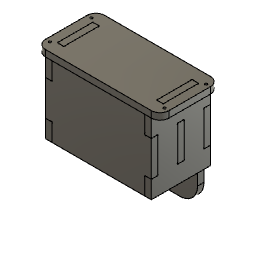
ArmorToolPocketHoleStation v2 (Autodesk Fusion 360 design; units mm, degrees)
Autodesk Fusion 360 part; units mm, degrees
sketch "Sketch1" plane through (0, 0, 0) normal (0, 1, 0) x (1, 0, 0)
  line L0 (0, 0) -> (266.7, 0)
  line L1 (266.7, 0) -> (266.7, -18.542)
  line L2 (266.7, -18.542) -> (0, -18.542)
  line L3 (0, -18.542) -> (0, 0)
  dimension "d1" = 266.7
  dimension "d2" = 18.542
  constraint horizontal L0
  constraint vertical L1
  constraint horizontal L2
  constraint vertical L3
  constraint coincident L0.start L3.end
  measures "d1" distance of L0.start L0.end
  measures "d2" distance of L0.start L2.end
extrude "Extrude1" add sketch "Sketch1" along normal blind 203.2 makes body 1 in component "Component"
sketch "Sketch2" plane through (0, 0, 18.542) normal (0, 0, 1) x (1, 0, 0)
  line L0 (0, 0) -> (266.7, 0)
  line L1 (266.7, 0) -> (266.7, 203.2)
  line L2 (266.7, 203.2) -> (0, 203.2)
  line L3 (0, 203.2) -> (0, 0)
  line L4 (0, 203.2) -> (0, 152.4) construction
  line L5 (266.7, 203.2) -> (266.7, 152.4) construction
  line L6 (0, 152.4) -> (-18.542, 152.4)
  line L7 (-18.542, 152.4) -> (-18.542, 50.8)
  line L8 (-18.542, 50.8) -> (0, 50.8)
  line L9 (0, 50.8) -> (0, 152.4)
  line L10 (266.7, 152.4) -> (285.242, 152.4)
  line L11 (285.242, 152.4) -> (285.242, 50.8)
  line L12 (285.242, 50.8) -> (266.7, 50.8)
  line L13 (266.7, 50.8) -> (266.7, 152.4)
  dimension "d5" = 50.8
  dimension "d7" = 50.8
  dimension "d8" = 18.542
  dimension "d9" = 101.6
  dimension "d10" = 18.542
  dimension "d11" = 101.6
  constraint coincident L2.end L3.start
  constraint perpendicular L2 L4
  constraint coincident L1.end L2.start
  constraint perpendicular L2 L5
  constraint horizontal L6
  constraint vertical L7
  constraint horizontal L8
  constraint vertical L9
  constraint horizontal L10
  constraint vertical L11
  constraint horizontal L12
  constraint vertical L13
  measures "d5" distance of L2.end L4.end
  measures "d7" distance of L1.end L5.end
  measures "d8" distance of L4.end L6.end
  measures "d9" distance of L4.end L8.end
  measures "d10" distance of L5.end L10.end
  measures "d11" distance of L5.end L12.end
extrude "Extrude2" add sketch "Sketch2" against normal up to surface (18.542 mm away) contours L3 L6 L7 L8 L9 | L1 L10 L11 L12 L13 bodies 1 in component "Component"
sketch "Sketch3" plane through (0, 0, 0) normal (-1, 0, 0) x (0, 0, 1)
  line L0 (0, 152.4) -> (18.542, 152.4)
  line L1 (18.542, 152.4) -> (18.542, 50.8)
  line L2 (18.542, 50.8) -> (0, 50.8)
  line L3 (0, 50.8) -> (0, 152.4)
  line L4 (94.234, 203.2) -> (94.234, 152.4)
  line L5 (94.234, 152.4) -> (75.692, 152.4)
  line L6 (75.692, 152.4) -> (75.692, 50.8)
  line L7 (75.692, 50.8) -> (94.234, 50.8)
  line L8 (94.234, 50.8) -> (94.234, 0)
  line L9 (94.234, 0) -> (-75.692, 0)
  line L10 (-75.692, 0) -> (-75.692, 50.8)
  line L11 (-75.692, 50.8) -> (-57.15, 50.8)
  line L12 (-57.15, 50.8) -> (-57.15, 152.4)
  line L13 (-57.15, 152.4) -> (-75.692, 152.4)
  line L14 (-75.692, 152.4) -> (-75.692, 203.2)
  line L15 (-75.692, 203.2) -> (94.234, 203.2)
  dimension "d15" = 50.8
  dimension "d16" = 18.542
  dimension "d17" = 101.6
  dimension "d18" = 18.542
  dimension "d19" = 169.926
  dimension "d20" = 18.542
  dimension "d21" = 101.6
  constraint coincident L0.end L1.start
  constraint perpendicular L0 L1
  constraint perpendicular L1 L2
  constraint coincident L0.start L3.end
  constraint perpendicular L0 L3
  constraint perpendicular L4 L5
  constraint perpendicular L5 L6
  constraint perpendicular L6 L7
  constraint perpendicular L7 L8
  constraint perpendicular L8 L9
  constraint perpendicular L9 L10
  constraint perpendicular L10 L11
  constraint perpendicular L9 L12
  constraint perpendicular L3 L13
  constraint perpendicular L13 L14
  measures "d15" distance of L4.start L4.end
  measures "d16" distance of L4.end L5.end
  measures "d17" distance of L5.end L6.end
  measures "d18" distance of L6.end L7.end
  measures "d19" distance of L8.end L9.end
  measures "d20" distance of L10.end L11.end
  measures "d21" distance of L11.end L12.end
extrude "Extrude1'" add sketch "Sketch3" along normal blind 18.542 separate body makes body 2 in component "Component'"
sketch "Sketch4" plane through (0, 0, -57.15) normal (0, 0, -1) x (-1, 0, 0)
  line L0 (0, 50.8) -> (18.542, 50.8)
  line L1 (18.542, 50.8) -> (18.542, 152.4)
  line L2 (18.542, 152.4) -> (0, 152.4)
  line L3 (0, 50.8) -> (0, -101.6)
  line L4 (0, -101.6) -> (-266.7, -101.6)
  line L5 (-266.7, -101.6) -> (-266.7, 50.8)
  line L6 (-266.7, 50.8) -> (-285.242, 50.8)
  line L7 (-285.242, 50.8) -> (-285.242, 152.4)
  line L8 (-285.242, 152.4) -> (-266.7, 152.4)
  line L9 (-266.7, 152.4) -> (-266.7, 203.2)
  line L10 (-266.7, 203.2) -> (0, 203.2)
  line L11 (0, 203.2) -> (0, 152.4)
  dimension "d24" = 152.4
  dimension "d25" = 266.7
  dimension "d26" = 18.542
  constraint coincident L0.start L3.start
  constraint perpendicular L0 L3
  constraint perpendicular L3 L4
  constraint perpendicular L4 L5
  constraint perpendicular L5 L6
  constraint perpendicular L6 L7
  constraint perpendicular L7 L8
  constraint perpendicular L8 L9
  constraint perpendicular L9 L10
  constraint coincident L2.end L11.end
  constraint perpendicular L2 L11
  measures "d24" distance of L0.start L3.end
  measures "d25" distance of L3.end L4.end
  measures "d26" distance of L5.end L6.end
extrude "Extrude1''" add sketch "Sketch4" along normal blind 18.542 separate body makes body 3 in component "Component''"
fillet "Fillet1" radius 50.8 2 edges at (266.7, -101.6, -66.421) (0, -101.6, -66.421) on bodies 3 in component "Component''"
sketch "Sketch5" plane through (-18.542, 0, 0) normal (-1, 0, 0) x (0, 0, 1)
  line L0 (18.542, 50.8) -> (0, 50.8)
  line L1 (0, 50.8) -> (0, 152.4)
  line L2 (0, 152.4) -> (18.542, 152.4)
  line L3 (18.542, 152.4) -> (18.542, 50.8)
  line L4 (-75.692, 203.2) -> (-75.692, 152.4)
  line L5 (-75.692, 152.4) -> (-57.15, 152.4)
  line L6 (-57.15, 152.4) -> (-57.15, 50.8)
  line L7 (-57.15, 50.8) -> (-75.692, 50.8)
  line L8 (-75.692, 50.8) -> (-75.692, 0)
  line L9 (-75.692, 0) -> (94.234, 0)
  line L10 (94.234, 0) -> (94.234, 50.8)
  line L11 (94.234, 50.8) -> (75.692, 50.8)
  line L12 (75.692, 50.8) -> (75.692, 152.4)
  line L13 (75.692, 152.4) -> (94.234, 152.4)
  line L14 (94.234, 152.4) -> (94.234, 203.2)
  line L15 (94.234, 203.2) -> (-75.692, 203.2)
  line L16 (60.071, 184.658) -> (-41.529, 184.658)
  line L17 (-41.529, 184.658) -> (-41.529, 221.742)
  line L18 (-41.529, 221.742) -> (60.071, 221.742)
  line L19 (60.071, 221.742) -> (60.071, 184.658)
  line L20 (60.071, 184.658) -> (-41.529, 221.742) construction
  line L21 (-41.529, 184.658) -> (60.071, 221.742) construction
  point P0 (9.271, 203.2)
  dimension "d31" = 101.6
  dimension "d32" = 37.084
  constraint horizontal L16
  constraint perpendicular L16 L17
  constraint parallel L16 L18
  constraint parallel L17 L19
  constraint coincident L20 P0
  constraint coincident L21 P0
  constraint midpoint L15 P0
  measures "d31" distance of L17.end L18.end
  measures "d32" distance of L16.end L17.end
extrude "Extrude2'" add sketch "Sketch5" against normal up to surface (18.542 mm away) contours L15 L17 L18 L19 bodies 2 in component "Component'"
sketch "Sketch6" plane through (0, 203.2, 0) normal (0, 1, 0) x (-1, 0, 0)
  line L0 (18.542, -41.529) -> (0, -41.529)
  line L1 (0, -75.692) -> (18.542, -75.692)
  line L2 (18.542, -75.692) -> (18.542, -41.529)
  line L3 (0, -75.692) -> (-285.242, -75.692)
  line L4 (-285.242, -75.692) -> (-285.242, -41.529)
  line L5 (-285.242, -41.529) -> (-266.7, -41.529)
  line L6 (-266.7, -41.529) -> (-266.7, 60.071)
  line L7 (-266.7, 60.071) -> (-285.242, 60.071)
  line L8 (-285.242, 60.071) -> (-285.242, 94.234)
  line L9 (-285.242, 94.234) -> (18.542, 94.234)
  line L10 (18.542, 94.234) -> (18.542, 60.071)
  line L11 (18.542, 60.071) -> (0, 60.071)
  line L12 (0, 60.071) -> (0, -41.529)
  dimension "d35" = 285.242
  dimension "d36" = 34.163
  dimension "d37" = 18.542
  dimension "d38" = 101.6
  dimension "d39" = 18.542
  dimension "d40" = 34.163
  dimension "d41" = 303.784
  constraint coincident L1.start L3.start
  constraint perpendicular L2 L3
  constraint perpendicular L3 L4
  constraint perpendicular L4 L5
  constraint perpendicular L5 L6
  constraint perpendicular L6 L7
  constraint perpendicular L7 L8
  constraint perpendicular L6 L9
  constraint perpendicular L9 L10
  constraint perpendicular L10 L11
  constraint coincident L0.end L12.end
  constraint perpendicular L0 L12
  measures "d35" distance of L1.start L3.end
  measures "d36" distance of L3.end L4.end
  measures "d37" distance of L4.end L5.end
  measures "d38" distance of L5.end L6.end
  measures "d39" distance of L6.end L7.end
  measures "d40" distance of L7.end L8.end
  measures "d41" distance of L8.end L9.end
sketch "Sketch7" plane through (0, 221.742, 0) normal (0, 1, 0) x (-1, 0, 0)
  line L0 (-285.242, -75.692) -> (18.542, -75.692)
  line L1 (18.542, -41.529) -> (0, -41.529)
  line L2 (0, -41.529) -> (0, 60.071)
  line L3 (0, 60.071) -> (18.542, 60.071)
  line L4 (18.542, 94.234) -> (-285.242, 94.234)
  line L5 (-285.242, 60.071) -> (-266.7, 60.071)
  line L6 (-266.7, 60.071) -> (-266.7, -41.529)
  line L7 (-266.7, -41.529) -> (-285.242, -41.529)
  line L8 (18.542, -41.529) -> (18.542, 60.071)
  line L9 (-285.242, -41.529) -> (-285.242, 60.071)
  line L10 (18.542, -75.692) -> (43.942, -75.692)
  line L11 (18.542, 94.234) -> (43.942, 94.234)
  line L12 (43.942, -75.692) -> (43.942, 94.234)
  line L13 (-285.242, -75.692) -> (-310.642, -75.692)
  line L14 (-285.242, 94.234) -> (-310.642, 94.234)
  line L15 (-310.642, 94.234) -> (-310.642, -75.692)
  dimension "d45" = 25.4
  constraint coincident L1.start L8.start
  constraint coincident L3.end L8.end
  constraint coincident L7.end L9.start
  constraint coincident L5.start L9.end
  constraint coincident L0.end L10.start
  constraint coincident L4.start L11.start
  constraint coincident L0.start L13.start
  constraint coincident L4.end L14.start
  measures "d45" distance of L4.start L11.end
extrude "Extrude1'''" add sketch "Sketch7" against normal blind 18.542 separate body makes body 4 in component "Component'''"
fillet "Fillet1'" radius 25.4 4 edges at (-43.942, 212.471, -75.692) (-43.942, 212.471, 94.234) (310.642, 212.471, -75.692) (310.642, 212.471, 94.234) on bodies 4 in component "Component'''"
ref_plane "WorkPlane1" through (266.7, 50.8, 0) normal (0, 0, 1) x (1, 0, 0)
sketch "Sketch8" plane through (266.7, 50.8, 0) normal (0, 0, 1) x (1, 0, 0)
  line L0 (0, -50.8) -> (0, 0) construction
  line L1 (18.542, 0) -> (0, 0) construction
  line L2 (0, 0) -> (2.2451, -2.2451) construction
  circle A0 centre (2.2451, -2.2451) radius 3.175
  dimension "d53" = 3.175
  constraint coincident L0.end L1.end
  constraint coincident L0.end A0
  measures "d53" distance of L0.end L2.end
sweep "Sweep1" cut kept parallel profiles "Sketch8" along 1 edges at (266.7, 50.8, 9.271) section 1 on bodies 1 bodies 1 in component "Component"
ref_plane "WorkPlane2" through (266.7, 152.4, 18.542) normal (0, 0, -1) x (-1, 0, 0)
sketch "Sketch9" plane through (266.7, 152.4, 18.542) normal (0, 0, -1) x (-1, 0, 0)
  line L0 (0, 0) -> (0, 50.8) construction
  line L1 (-18.542, 0) -> (0, 0) construction
  line L2 (0, 0) -> (-2.2451, 2.2451) construction
  circle A0 centre (-2.2451, 2.2451) radius 3.175
  dimension "d61" = 3.175
  constraint coincident L0.start L1.end
  constraint coincident L0.start A0
  measures "d61" distance of L0.start L2.end
sweep "Sweep2" cut kept parallel profiles "Sketch9" along 1 edges at (266.7, 152.4, 9.271) section 1 on bodies 1 bodies 1 in component "Component"
ref_plane "WorkPlane3" through (0, 50.8, 18.542) normal (0, 0, -1) x (-1, 0, 0)
sketch "Sketch10" plane through (0, 50.8, 18.542) normal (0, 0, -1) x (-1, 0, 0)
  line L0 (0, -50.8) -> (0, 0) construction
  line L1 (18.542, 0) -> (0, 0) construction
  line L2 (0, 0) -> (2.2451, -2.2451) construction
  circle A0 centre (2.2451, -2.2451) radius 3.175
  dimension "d69" = 3.175
  constraint coincident L0.end L1.end
  constraint coincident L0.end A0
  measures "d69" distance of L0.end L2.end
sweep "Sweep3" cut kept parallel profiles "Sketch10" along 1 edges at (0, 50.8, 9.271) section 1 on bodies 1 bodies 1 in component "Component"
ref_plane "WorkPlane4" through (0, 152.4, 0) normal (0, 0, 1) x (1, 0, 0)
sketch "Sketch11" plane through (0, 152.4, 0) normal (0, 0, 1) x (1, 0, 0)
  line L0 (0, 0) -> (0, 50.8) construction
  line L1 (0, 0) -> (-18.542, 0) construction
  line L2 (0, 0) -> (-2.2451, 2.2451) construction
  circle A0 centre (-2.2451, 2.2451) radius 3.175
  dimension "d77" = 3.175
  constraint coincident L0.start L1.start
  constraint coincident L0.start A0
  measures "d77" distance of L0.start L2.end
sweep "Sweep4" cut kept parallel profiles "Sketch11" along 1 edges at (0, 152.4, 9.271) section 1 on bodies 1 bodies 1 in component "Component"
ref_plane "WorkPlane5" through (-18.542, 203.2, -41.529) normal (1, 0, 0) x (0, 1, 0)
sketch "Sketch12" plane through (-18.542, 203.2, -41.529) normal (1, 0, 0) x (0, 1, 0)
  line L0 (0, -34.163) -> (0, 0) construction
  line L1 (18.542, 0) -> (0, 0) construction
  line L2 (0, 0) -> (2.2451, -2.2451) construction
  circle A0 centre (2.2451, -2.2451) radius 3.175
  dimension "d85" = 3.175
  constraint coincident L0.end L1.end
  constraint coincident L0.end A0
  measures "d85" distance of L0.end L2.end
sweep "Sweep1'" cut kept parallel profiles "Sketch12" along 1 edges at (-9.271, 203.2, -41.529) section 1 on bodies 2 bodies 2 in component "Component'"
ref_plane "WorkPlane6" through (0, 50.8, -57.15) normal (-1, 0, 0) x (0, -1, 0)
sketch "Sketch13" plane through (0, 50.8, -57.15) normal (-1, 0, 0) x (0, -1, 0)
  line L0 (0, 0) -> (-101.6, 0) construction
  line L1 (0, -18.542) -> (0, 0) construction
  line L2 (0, 0) -> (-2.2451, -2.2451) construction
  circle A0 centre (-2.2451, -2.2451) radius 3.175
  dimension "d93" = 3.175
  constraint coincident L0.start L1.end
  constraint coincident L0.start A0
  measures "d93" distance of L0.start L2.end
sweep "Sweep2'" cut kept parallel profiles "Sketch13" along 1 edges at (-9.271, 50.8, -57.15) section 1 on bodies 2 bodies 2 in component "Component'"
ref_plane "WorkPlane7" through (0, 50.8, 18.542) normal (-1, 0, 0) x (0, -1, 0)
sketch "Sketch14" plane through (0, 50.8, 18.542) normal (-1, 0, 0) x (0, -1, 0)
  line L0 (0, 0) -> (0, -18.542) construction
  line L1 (-101.6, 0) -> (0, 0) construction
  line L2 (0, 0) -> (-2.2451, -2.2451) construction
  circle A0 centre (-2.2451, -2.2451) radius 3.175
  dimension "d101" = 3.175
  constraint coincident L0.start L1.end
  constraint coincident L0.start A0
  measures "d101" distance of L0.start L2.end
sweep "Sweep3'" cut kept parallel profiles "Sketch14" along 1 edges at (-9.271, 50.8, 18.542) section 1 on bodies 2 bodies 2 in component "Component'"
ref_plane "WorkPlane8" through (0, 152.4, -57.15) normal (-1, 0, 0) x (0, -1, 0)
sketch "Sketch15" plane through (0, 152.4, -57.15) normal (-1, 0, 0) x (0, -1, 0)
  line L0 (0, 0) -> (0, -18.542) construction
  line L1 (97.1099, 0) -> (0, 0) construction
  line L2 (0, 0) -> (2.2451, -2.2451) construction
  circle A0 centre (2.2451, -2.2451) radius 3.175
  dimension "d109" = 3.175
  constraint coincident L0.start L1.end
  constraint coincident L0.start A0
  measures "d109" distance of L0.start L2.end
sweep "Sweep4'" cut kept parallel profiles "Sketch15" along 1 edges at (-9.271, 152.4, -57.15) section 1 on bodies 2 bodies 2 in component "Component'"
ref_plane "WorkPlane9" through (0, 152.4, 18.542) normal (-1, 0, 0) x (0, -1, 0)
sketch "Sketch16" plane through (0, 152.4, 18.542) normal (-1, 0, 0) x (0, -1, 0)
  line L0 (0, -18.542) -> (0, 0) construction
  line L1 (0, 0) -> (97.1099, 0) construction
  line L2 (0, 0) -> (2.2451, -2.2451) construction
  circle A0 centre (2.2451, -2.2451) radius 3.175
  dimension "d117" = 3.175
  constraint coincident L0.end L1.start
  constraint coincident L0.end A0
  measures "d117" distance of L0.end L2.end
sweep "Sweep5" cut kept parallel profiles "Sketch16" along 1 edges at (-9.271, 152.4, 18.542) section 1 on bodies 2 bodies 2 in component "Component'"
ref_plane "WorkPlane10" through (0, 203.2, 60.071) normal (-1, 0, 0) x (0, -1, 0)
sketch "Sketch17" plane through (0, 203.2, 60.071) normal (-1, 0, 0) x (0, -1, 0)
  line L0 (0, 34.163) -> (0, 0) construction
  line L1 (-18.542, 0) -> (0, 0) construction
  line L2 (0, 0) -> (-2.2451, 2.2451) construction
  circle A0 centre (-2.2451, 2.2451) radius 3.175
  dimension "d125" = 3.175
  constraint coincident L0.end L1.end
  constraint coincident L0.end A0
  measures "d125" distance of L0.end L2.end
sweep "Sweep6" cut kept parallel profiles "Sketch17" along 1 edges at (-9.271, 203.2, 60.071) section 1 on bodies 2 bodies 2 in component "Component'"
ref_plane "WorkPlane11" through (0, 50.8, 0) normal (-1, 0, 0) x (0, -1, 0)
sketch "Sketch18" plane through (0, 50.8, 0) normal (-1, 0, 0) x (0, -1, 0)
  line L0 (0, 14.0519) -> (0, 0) construction
  line L1 (0, 0) -> (-101.6, 0) construction
  line L2 (0, 0) -> (-2.2451, 2.2451) construction
  circle A0 centre (-2.2451, 2.2451) radius 3.175
  dimension "d133" = 3.175
  constraint coincident L0.end L1.start
  constraint coincident L0.end A0
  measures "d133" distance of L0.end L2.end
sweep "Sweep7" cut kept parallel profiles "Sketch18" along 1 edges at (-9.271, 50.8, 0) section 1 on bodies 2 bodies 2 in component "Component'"
ref_plane "WorkPlane12" through (0, 50.8, 75.692) normal (-1, 0, 0) x (0, -1, 0)
sketch "Sketch19" plane through (0, 50.8, 75.692) normal (-1, 0, 0) x (0, -1, 0)
  line L0 (0, 0) -> (0, 18.542) construction
  line L1 (-101.6, 0) -> (0, 0) construction
  line L2 (0, 0) -> (-2.2451, 2.2451) construction
  circle A0 centre (-2.2451, 2.2451) radius 3.175
  dimension "d141" = 3.175
  constraint coincident L0.start L1.end
  constraint coincident L0.start A0
  measures "d141" distance of L0.start L2.end
sweep "Sweep8" cut kept parallel profiles "Sketch19" along 1 edges at (-9.271, 50.8, 75.692) section 1 on bodies 2 bodies 2 in component "Component'"
ref_plane "WorkPlane13" through (0, 152.4, 0) normal (-1, 0, 0) x (0, -1, 0)
sketch "Sketch20" plane through (0, 152.4, 0) normal (-1, 0, 0) x (0, -1, 0)
  line L0 (97.1099, 0) -> (0, 0) construction
  line L1 (0, 0) -> (0, 14.0519) construction
  line L2 (0, 0) -> (2.2451, 2.2451) construction
  circle A0 centre (2.2451, 2.2451) radius 3.175
  dimension "d149" = 3.175
  constraint coincident L0.end L1.start
  constraint coincident L0.end A0
  measures "d149" distance of L0.end L2.end
sweep "Sweep9" cut kept parallel profiles "Sketch20" along 1 edges at (-9.271, 152.4, 0) section 1 on bodies 2 bodies 2 in component "Component'"
ref_plane "WorkPlane14" through (0, 152.4, 75.692) normal (-1, 0, 0) x (0, -1, 0)
sketch "Sketch21" plane through (0, 152.4, 75.692) normal (-1, 0, 0) x (0, -1, 0)
  line L0 (0, 0) -> (97.1099, 0) construction
  line L1 (0, 18.542) -> (0, 0) construction
  line L2 (0, 0) -> (2.2451, 2.2451) construction
  circle A0 centre (2.2451, 2.2451) radius 3.175
  dimension "d157" = 3.175
  constraint coincident L0.start L1.end
  constraint coincident L0.start A0
  measures "d157" distance of L0.start L2.end
sweep "Sweep10" cut kept parallel profiles "Sketch21" along 1 edges at (-9.271, 152.4, 75.692) section 1 on bodies 2 bodies 2 in component "Component'"
ref_plane "WorkPlane15" through (0, 50.8, -57.15) normal (0, 0, -1) x (-1, 0, 0)
sketch "Sketch22" plane through (0, 50.8, -57.15) normal (0, 0, -1) x (-1, 0, 0)
  line L0 (0, 0) -> (18.542, 0) construction
  line L1 (0, 0) -> (0, -101.6) construction
  line L2 (0, 0) -> (2.2451, -2.2451) construction
  circle A0 centre (2.2451, -2.2451) radius 3.175
  dimension "d165" = 3.175
  constraint coincident L0.start L1.start
  constraint coincident L0.start A0
  measures "d165" distance of L0.start L2.end
sweep "Sweep1''" cut kept parallel profiles "Sketch22" along 1 edges at (0, 50.8, -66.421) section 1 on bodies 3 bodies 3 in component "Component''"
ref_plane "WorkPlane16" through (0, 152.4, -57.15) normal (0, 0, -1) x (-1, 0, 0)
sketch "Sketch23" plane through (0, 152.4, -57.15) normal (0, 0, -1) x (-1, 0, 0)
  line L0 (18.542, 0) -> (0, 0) construction
  line L1 (0, 50.8) -> (0, 0) construction
  line L2 (0, 0) -> (2.2451, 2.2451) construction
  circle A0 centre (2.2451, 2.2451) radius 3.175
  dimension "d173" = 3.175
  constraint coincident L0.end L1.end
  constraint coincident L0.end A0
  measures "d173" distance of L0.end L2.end
sweep "Sweep2''" cut kept parallel profiles "Sketch23" along 1 edges at (0, 152.4, -66.421) section 1 on bodies 3 bodies 3 in component "Component''"
ref_plane "WorkPlane17" through (266.7, 152.4, -57.15) normal (0, 0, -1) x (-1, 0, 0)
sketch "Sketch24" plane through (266.7, 152.4, -57.15) normal (0, 0, -1) x (-1, 0, 0)
  line L0 (0, 0) -> (0, 50.8) construction
  line L1 (-18.542, 0) -> (0, 0) construction
  line L2 (0, 0) -> (-2.2451, 2.2451) construction
  circle A0 centre (-2.2451, 2.2451) radius 3.175
  dimension "d181" = 3.175
  constraint coincident L0.start L1.end
  constraint coincident L0.start A0
  measures "d181" distance of L0.start L2.end
sweep "Sweep3''" cut kept parallel profiles "Sketch24" along 1 edges at (266.7, 152.4, -66.421) section 1 on bodies 3 bodies 3 in component "Component''"
ref_plane "WorkPlane18" through (266.7, 50.8, -57.15) normal (0, 0, -1) x (-1, 0, 0)
sketch "Sketch25" plane through (266.7, 50.8, -57.15) normal (0, 0, -1) x (-1, 0, 0)
  line L0 (0, 0) -> (-18.542, 0) construction
  line L1 (0, -101.6) -> (0, 0) construction
  line L2 (0, 0) -> (-2.2451, -2.2451) construction
  circle A0 centre (-2.2451, -2.2451) radius 3.175
  dimension "d189" = 3.175
  constraint coincident L0.start L1.end
  constraint coincident L0.start A0
  measures "d189" distance of L0.start L2.end
sweep "Sweep4''" cut kept parallel profiles "Sketch25" along 1 edges at (266.7, 50.8, -66.421) section 1 on bodies 3 bodies 3 in component "Component''"
ref_plane "WorkPlane19" through (-18.542, 221.742, 60.071) normal (0, -1, 0) x (1, 0, 0)
sketch "Sketch26" plane through (-18.542, 221.742, 60.071) normal (0, -1, 0) x (1, 0, 0)
  line L0 (0, 0) -> (0, -101.6) construction
  line L1 (18.542, 0) -> (0, 0) construction
  line L2 (0, 0) -> (2.2451, -2.2451) construction
  circle A0 centre (2.2451, -2.2451) radius 3.175
  dimension "d197" = 3.175
  constraint coincident L0.start L1.end
  constraint coincident L0.start A0
  measures "d197" distance of L0.start L2.end
sweep "Sweep1'''" cut kept parallel profiles "Sketch26" along 1 edges at (-18.542, 212.471, 60.071) section 1 on bodies 4 bodies 4 in component "Component'''"
ref_plane "WorkPlane20" through (266.7, 221.742, 60.071) normal (0, -1, 0) x (1, 0, 0)
sketch "Sketch27" plane through (266.7, 221.742, 60.071) normal (0, -1, 0) x (1, 0, 0)
  line L0 (0, 0) -> (0, -101.6) construction
  line L1 (18.542, 0) -> (0, 0) construction
  line L2 (0, 0) -> (2.2451, -2.2451) construction
  circle A0 centre (2.2451, -2.2451) radius 3.175
  dimension "d205" = 3.175
  constraint coincident L0.start L1.end
  constraint coincident L0.start A0
  measures "d205" distance of L0.start L2.end
sweep "Sweep2'''" cut kept parallel profiles "Sketch27" along 1 edges at (266.7, 212.471, 60.071) section 1 on bodies 4 bodies 4 in component "Component'''"
ref_plane "WorkPlane21" through (266.7, 221.742, -41.529) normal (0, -1, 0) x (1, 0, 0)
sketch "Sketch28" plane through (266.7, 221.742, -41.529) normal (0, -1, 0) x (1, 0, 0)
  line L0 (0, 0) -> (18.542, 0) construction
  line L1 (0, 97.1099) -> (0, 0) construction
  line L2 (0, 0) -> (2.2451, 2.2451) construction
  circle A0 centre (2.2451, 2.2451) radius 3.175
  dimension "d213" = 3.175
  constraint coincident L0.start L1.end
  constraint coincident L0.start A0
  measures "d213" distance of L0.start L2.end
sweep "Sweep3'''" cut kept parallel profiles "Sketch28" along 1 edges at (266.7, 212.471, -41.529) section 1 on bodies 4 bodies 4 in component "Component'''"
ref_plane "WorkPlane22" through (285.242, 221.742, -41.529) normal (0, -1, 0) x (1, 0, 0)
sketch "Sketch29" plane through (285.242, 221.742, -41.529) normal (0, -1, 0) x (1, 0, 0)
  line L0 (0, 0) -> (-14.0519, 0) construction
  line L1 (0, 101.6) -> (0, 0) construction
  line L2 (0, 0) -> (-2.2451, 2.2451) construction
  circle A0 centre (-2.2451, 2.2451) radius 3.175
  dimension "d221" = 3.175
  constraint coincident L0.start L1.end
  constraint coincident L0.start A0
  measures "d221" distance of L0.start L2.end
sweep "Sweep4'''" cut kept parallel profiles "Sketch29" along 1 edges at (285.242, 212.471, -41.529) section 1 on bodies 4 bodies 4 in component "Component'''"
ref_plane "WorkPlane23" through (285.242, 221.742, 60.071) normal (0, -1, 0) x (1, 0, 0)
sketch "Sketch30" plane through (285.242, 221.742, 60.071) normal (0, -1, 0) x (1, 0, 0)
  line L0 (0, 0) -> (-14.0519, 0) construction
  line L1 (0, -97.1099) -> (0, 0) construction
  line L2 (0, 0) -> (-2.2451, -2.2451) construction
  circle A0 centre (-2.2451, -2.2451) radius 3.175
  dimension "d229" = 3.175
  constraint coincident L0.start L1.end
  constraint coincident L0.start A0
  measures "d229" distance of L0.start L2.end
sweep "Sweep5'" cut kept parallel profiles "Sketch30" along 1 edges at (285.242, 212.471, 60.071) section 1 on bodies 4 bodies 4 in component "Component'''"
ref_plane "WorkPlane24" through (-18.542, 221.742, -41.529) normal (0, -1, 0) x (1, 0, 0)
sketch "Sketch31" plane through (-18.542, 221.742, -41.529) normal (0, -1, 0) x (1, 0, 0)
  line L0 (0, 0) -> (18.542, 0) construction
  line L1 (0, 97.1099) -> (0, 0) construction
  line L2 (0, 0) -> (2.2451, 2.2451) construction
  circle A0 centre (2.2451, 2.2451) radius 3.175
  dimension "d237" = 3.175
  constraint coincident L0.start L1.end
  constraint coincident L0.start A0
  measures "d237" distance of L0.start L2.end
sweep "Sweep6'" cut kept parallel profiles "Sketch31" along 1 edges at (-18.542, 212.471, -41.529) section 1 on bodies 4 bodies 4 in component "Component'''"
ref_plane "WorkPlane25" through (0, 221.742, 60.071) normal (0, -1, 0) x (1, 0, 0)
sketch "Sketch32" plane through (0, 221.742, 60.071) normal (0, -1, 0) x (1, 0, 0)
  line L0 (0, 0) -> (-14.0519, 0) construction
  line L1 (0, -101.6) -> (0, 0) construction
  line L2 (0, 0) -> (-2.2451, -2.2451) construction
  circle A0 centre (-2.2451, -2.2451) radius 3.175
  dimension "d245" = 3.175
  constraint coincident L0.start L1.end
  constraint coincident L0.start A0
  measures "d245" distance of L0.start L2.end
sweep "Sweep7'" cut kept parallel profiles "Sketch32" along 1 edges at (0, 212.471, 60.071) section 1 on bodies 4 bodies 4 in component "Component'''"
ref_plane "WorkPlane26" through (0, 221.742, -41.529) normal (0, -1, 0) x (1, 0, 0)
sketch "Sketch33" plane through (0, 221.742, -41.529) normal (0, -1, 0) x (1, 0, 0)
  line L0 (0, 0) -> (-14.0519, 0) construction
  line L1 (0, 97.1099) -> (0, 0) construction
  line L2 (0, 0) -> (-2.2451, 2.2451) construction
  circle A0 centre (-2.2451, 2.2451) radius 3.175
  dimension "d253" = 3.175
  constraint coincident L0.start L1.end
  constraint coincident L0.start A0
  measures "d253" distance of L0.start L2.end
sweep "Sweep8'" cut kept parallel profiles "Sketch33" along 1 edges at (0, 212.471, -41.529) section 1 on bodies 4 bodies 4 in component "Component'''"
sketch "Sketch34" plane through (0, 221.742, 0) normal (0, 1, 0) x (-1, 0, 0)
  arc A0 (0, -37.0389) -> (4.4901, -41.529) centre (2.2451, -39.2839) ccw
  line L0 (0, -37.0389) -> (0, 55.5809)
  arc A1 (4.4901, 60.071) -> (0, 55.5809) centre (2.2451, 57.8259) ccw
  line L1 (4.4901, 60.071) -> (14.0519, 60.071)
  arc A2 (18.542, 55.5809) -> (14.0519, 60.071) centre (16.2969, 57.8259) ccw
  line L2 (18.542, 55.5809) -> (18.542, -37.0389)
  arc A3 (14.0519, -41.529) -> (18.542, -37.0389) centre (16.2969, -39.2839) ccw
  line L3 (14.0519, -41.529) -> (4.4901, -41.529)
  arc A4 (-285.242, 94.234) -> (-310.642, 68.834) centre (-285.242, 68.834) ccw
  line L4 (-310.642, 68.834) -> (-310.642, -50.292)
  arc A5 (-310.642, -50.292) -> (-285.242, -75.692) centre (-285.242, -50.292) ccw
  line L5 (-285.242, -75.692) -> (18.542, -75.692)
  arc A6 (18.542, -75.692) -> (43.942, -50.292) centre (18.542, -50.292) ccw
  line L6 (43.942, -50.292) -> (43.942, 68.834)
  arc A7 (43.942, 68.834) -> (18.542, 94.234) centre (18.542, 68.834) ccw
  line L7 (18.542, 94.234) -> (-285.242, 94.234)
  arc A8 (-280.7519, 60.071) -> (-285.242, 55.5809) centre (-282.9969, 57.8259) ccw
  line L8 (-280.7519, 60.071) -> (-271.1901, 60.071)
  arc A9 (-266.7, 55.5809) -> (-271.1901, 60.071) centre (-268.9451, 57.8259) ccw
  line L9 (-266.7, 55.5809) -> (-266.7, -37.0389)
  arc A10 (-271.1901, -41.529) -> (-266.7, -37.0389) centre (-268.9451, -39.2839) ccw
  line L10 (-271.1901, -41.529) -> (-280.7519, -41.529)
  arc A11 (-285.242, -37.0389) -> (-280.7519, -41.529) centre (-282.9969, -39.2839) ccw
  line L11 (-285.242, -37.0389) -> (-285.242, 55.5809)
  line L12 (43.942, -50.292) -> (31.242, -50.292) construction
  line L13 (43.942, 68.834) -> (31.242, 68.834) construction
  line L14 (-310.642, -50.292) -> (-297.942, -50.292) construction
  line L15 (-310.642, 68.834) -> (-297.942, 68.834) construction
  circle A12 centre (-297.942, -50.292) radius 3.429
  circle A13 centre (-297.942, 68.834) radius 3.429
  circle A14 centre (31.242, -50.292) radius 3.429
  circle A15 centre (31.242, 68.834) radius 3.429
  dimension "d260" = 12.7
  dimension "d261" = 12.7
  dimension "d262" = 12.7
  dimension "d263" = 12.7
  dimension "d264" = 6.858
  dimension "d265" = 6.858
  dimension "d266" = 6.858
  dimension "d267" = 6.858
  constraint coincident A6.end L6.start
  constraint perpendicular L6 L12
  constraint coincident L6.end A7.start
  constraint perpendicular L6 L13
  constraint coincident L4.end A5.start
  constraint perpendicular L4 L14
  constraint coincident A4.end L4.start
  constraint perpendicular L4 L15
  constraint coincident L14.end A12.centre
  constraint coincident L15.end A13.centre
  constraint coincident L12.end A14.centre
  constraint coincident L13.end A15.centre
  measures "d260" distance of A6.end L12.end
  measures "d261" distance of L6.end L13.end
  measures "d262" distance of L4.end L14.end
  measures "d263" distance of A4.end L15.end
  measures "d264" diameter of A12
  measures "d265" diameter of A13
  measures "d266" diameter of A14
  measures "d267" diameter of A15
extrude "Extrude2''" cut sketch "Sketch34" against normal up to surface (18.542 mm away) contours A12 | A13 | A14 | A15 bodies 4 in component "Component'''"
component "Component" placed x (1, 0, 0) y (0, 1, 0) z (0, 0, 1) at (0, 0, 0)
component "Component'" placed x (1, 0, 0) y (0, 1, 0) z (0, 0, 1) at (0, 0, 0)
component "Component" placed x (1, 0, 0) y (0, 1, 0) z (0, 0, 1) at (0, 0, 75.692)
component "Component'" placed x (1, 0, 0) y (0, 1, 0) z (0, 0, 1) at (285.242, 0, 0)
component "Component''" placed x (1, 0, 0) y (0, 1, 0) z (0, 0, 1) at (0, 0, 0)
component "Component'''" placed x (1, 0, 0) y (0, 1, 0) z (0, 0, 1) at (0, 0, 0)
equation "d19 = 2.25 in + 2.25 in + ( 0.73 * 3 ) * 1 in"
equation "d32 = ( 0.73 * 2 ) * 1 in"
equation "d35 = 10.5 in + 0.73 in"
equation "d41 = 10.5 in + ( 0.73 * 2 ) * 1 in"
equation "d53 = 0.25 in / 2 + 0.00 in"
equation "d61 = 0.25 in / 2 + 0.00 in"
equation "d69 = 0.25 in / 2 + 0.00 in"
equation "d77 = 0.25 in / 2 + 0.00 in"
equation "d85 = 0.25 in / 2 + 0.00 in"
equation "d93 = 0.25 in / 2 + 0.00 in"
equation "d101 = 0.25 in / 2 + 0.00 in"
equation "d109 = 0.25 in / 2 + 0.00 in"
equation "d117 = 0.25 in / 2 + 0.00 in"
equation "d125 = 0.25 in / 2 + 0.00 in"
equation "d133 = 0.25 in / 2 + 0.00 in"
equation "d141 = 0.25 in / 2 + 0.00 in"
equation "d149 = 0.25 in / 2 + 0.00 in"
equation "d157 = 0.25 in / 2 + 0.00 in"
equation "d165 = 0.25 in / 2 + 0.00 in"
equation "d173 = 0.25 in / 2 + 0.00 in"
equation "d181 = 0.25 in / 2 + 0.00 in"
equation "d189 = 0.25 in / 2 + 0.00 in"
equation "d197 = 0.25 in / 2 + 0.00 in"
equation "d205 = 0.25 in / 2 + 0.00 in"
equation "d213 = 0.25 in / 2 + 0.00 in"
equation "d221 = 0.25 in / 2 + 0.00 in"
equation "d229 = 0.25 in / 2 + 0.00 in"
equation "d237 = 0.25 in / 2 + 0.00 in"
equation "d245 = 0.25 in / 2 + 0.00 in"
equation "d253 = 0.25 in / 2 + 0.00 in"
